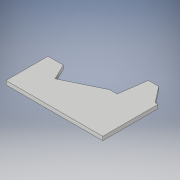
# Autodesk Inventor part: Side Panel
Saved by Autodesk Inventor 2017 (Build 210142000, 142)
## iProperties
Created: 2019-03-08
Part Number: Side Panel
Material: Generic
Document SubType Name: Modeling
Designer: Mitch
Density: 1 g/cm^3
Appearance: Default
Author: Mitch
Autodesk Inventor part; units mm, degrees
ref_plane "YZ Plane" through (0, 0, 0) normal (1, 0, 0) x (0, 1, 0)
ref_plane "XZ Plane" through (0, 0, 0) normal (0, 1, 0) x (-1, 0, 0)
ref_plane "XY Plane" through (0, 0, 0) normal (0, 0, 1) x (1, 0, 0)
sketch "Sketch1" plane through (0, 0, 0) normal (0, 1, 0) x (-1, 0, 0)
  line L0 (0, 0) -> (482.6, 0)
  line L1 (482.6, 0) -> (482.6, -209.55)
  line L2 (482.6, -209.55) -> (406.4, -209.55)
  line L3 (406.4, -209.55) -> (367.4288, -129.6472)
  line L4 (367.4288, -129.6472) -> (184.7939, -218.7242)
  line L5 (184.7939, -218.7242) -> (146.6939, -218.7242)
  line L6 (146.6939, -218.7242) -> (127.4536, -355.6254)
  line L7 (127.4536, -355.6254) -> (76.6536, -355.6254)
  line L8 (76.6536, -355.6254) -> (14.1024, -275.5635)
  line L9 (14.1024, -275.5635) -> (0, -275.5635)
  line L10 (0, 0) -> (0, -275.5635)
  point P0 (438.8308, 0)
  point P1 (482.6, -106.5112)
  dimension "d22" = 98
  dimension "d23" = 154
  dimension "d26" = 76.2
  dimension "d27" = 128
  dimension "d29" = 355.6254
  dimension "d30" = 88.9
  dimension "d33" = 203.2
  dimension "d34" = 38.1
  dimension "d35" = 50.8
  dimension "d36" = 101.6
  dimension "d37" = 138.2466
  dimension "d38" = 209.55
  dimension "d39" = 482.6
  constraints: 22 end point, 3 horizontal, 3 perpendicular, 2 point on line, 1 parallel, 1 vertical
  measures "d22" angle of L6 L7
  measures "d23" angle of L4 L5
  measures "d26" distance of L1.end L2.end
  measures "d27" angle of L8 L9
  measures "d29" distance between parallel lines of L0 L7
  measures "d30" distance of L2.end L3.end
  measures "d33" distance of L3.end L4.end
  measures "d34" distance of L4.end L5.end
  measures "d35" distance of L6.end L7.end
  measures "d36" distance of L7.end L8.end
  measures "d37" distance of L5.end L6.end
  measures "d38" distance of L0.end L1.end
  measures "d39" distance of L0.start L0.end
extrude "Extrusion1" add sketch "Sketch1" along normal blind 19.05
body "Solid1"
